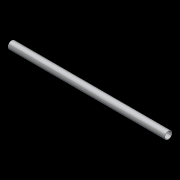
# Autodesk Inventor part: TuboEstructura
Saved by Autodesk Inventor 2.016 (Build 200138000, 138)
## iProperties
Created: 2014-07-11
Part Number: TuboEstructura
Material: Aluminum 6061
Document SubType Name: Modeling
Designer: Jose
Density: 2.71 g/cm^3
Appearance: Aluminum - Flat
Mass: 39.3334 g
Surface Area: 291.163 cm^2
Volume: 14.5142 cm^3
Author: Jose
Autodesk Inventor part; units mm, degrees
ref_plane "YZ Plane" through (0, 0, 0) normal (1, 0, 0) x (0, 1, 0)
ref_plane "XZ Plane" through (0, 0, 0) normal (0, 1, 0) x (-1, 0, 0)
ref_plane "XY Plane" through (0, 0, 0) normal (0, 0, 1) x (1, 0, 0)
sketch "Sketch1" plane through (0, 0, 0) normal (1, 0, 0) x (0, 1, 0)
  circle A0 centre (0, 0) radius 8
  circle A1 centre (0, 0) radius 7
  dimension "d0" = 16
  dimension "d1" = 1
  constraints: 2 centre point, 2 coincident
  measures "d0" diameter of A0
  measures "d1" radial gap between concentric circles of A0 A1
extrude "Extrusion1" add sketch "Sketch1" along normal blind 330
body "Solid1"
